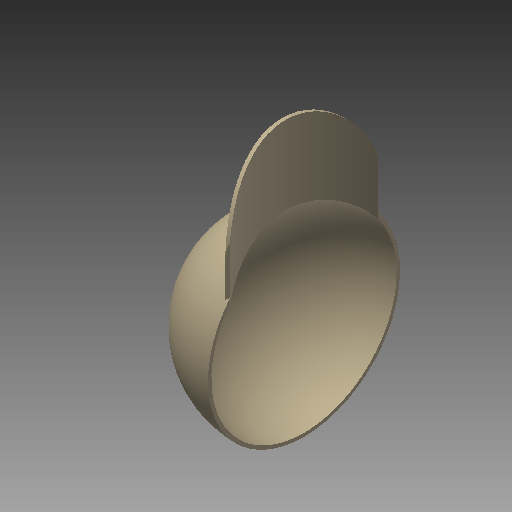
# Autodesk Inventor part: 3D HUMAN
Saved by Autodesk Inventor 2022 (Build 260153000, 153)
## iProperties
Category: PART
Part Number: 3D HUMAN
Document SubType Name: Modeling
Created: 2003-07-26
Designer: M.F.
Manufacturer: Standard
Standards Organization: Custom
Catalog Web Link: www.apollocanard.com
Density: 1 g/cm^3
Material: Generic
Appearance: Beige
Control State: 0
Master: False
Checked Out: False
Shininess: 64.0
Length Units: 11272
Angle Units: 11279
Time Units: 11290
Mass Units: 11286
Length Display Precision: 3
Angle Display Precision: 2
Compacted: True
Density: 0.0
Volumn: 0.0
Area: 0.0
PropertySet Name: Model Information
Title: iMan
Author: M.F.
Autodesk Inventor part; units mm, degrees
sketch "Sketch2" plane through (0, 0, 0) normal (0, 0, 1) x (1, 0, 0)
  line L0 (96.9814, 0) -> (100.5374, 0)
  arc A0 (100.5374, 0) -> (0, 100.5374) centre (0, 0) ccw
  line L1 (0, 100.5374) -> (0, 96.9814)
  arc A1 (96.9814, 0) -> (0, 96.9814) centre (0, 0) ccw
  dimension "d25" = 96.9814
  dimension "d26" = 3.556
  constraints: 4 end point, 4 point on circle, 2 centre point, 2 coincident, 2 point on line, 1 horizontal, 1 perpendicular
  measures "d25" radius of A1
  measures "d26" distance of L0.start L0.end
revolve "Revolution1" add sketch "Sketch2" angle 360 about axis through (0, 100.5374, 0) along (0, -1, 0)
ref_plane "Work Plane1" through (0, 0, 100.5374) normal (0, 0, 1) x (1, 0, 0)
ref_plane "Work Plane2" through (0, 0, 197.5188) normal (0, 0, 1) x (1, 0, 0)
sketch "Sketch4" plane through (0, 0, 197.5188) normal (0, 0, 1) x (1, 0, 0)
  line L0 (-96.9814, 0) -> (96.9814, 0) projected
  arc A0 (0, 19.3963) -> (-77.5851, 0) centre (0, -145.4721) ccw
  arc A1 (0, 22.9523) -> (-79.2585, 3.1376) centre (0, -145.4721) ccw
  line L1 (0, 19.3963) -> (0, 22.9523)
  line L2 (-79.2585, 3.1376) -> (-77.5851, 0)
  point P0 (0, 0)
  dimension "d30" = 19.3963
  dimension "d31" = 19.3963
  dimension "d32" = 3.556
  constraints: 5 point on circle, 4 end point, 2 centre point, 2 vertical alignment, 1 midpoint, 1 perpendicular, 1 point on line
  measures "d30" distance from line of A0.start L0
  measures "d31" distance of L0.start L2.end
  measures "d32" distance of L1.start L1.end
extrude "Extrusion1" add sketch "Sketch4" against normal up to next
mirror "Mirror1" about plane through (0, 19.3963, 197.5188) normal (1, 0, 0) of "Extrusion1"
sketch "Sketch5" plane through (0, 0, 197.5188) normal (0, 0, 1) x (1, 0, 0)
  arc A0 (77.5851, 0) -> (-77.5851, 0) centre (0, -145.4721) ccw projected
  line L0 (-77.5851, 0) -> (77.5851, 0)
  constraints: 2 end point, 1 horizontal
extrude "Extrusion2" cut sketch "Sketch5" against normal up to surface (197.5188 mm away)
sketch "Sketch6" plane through (0, 0, 0) normal (0, 1, 0) x (-1, 0, 0)
  arc A0 (79.2585, 97.8824) -> (-79.2585, 97.8824) centre (0, 97.8824) ccw
  spline S0 degree 3 poles (79.2585, 61.7739) (78.7898, 62.3626) (78.3161, 62.9424) (76.2018, 65.4662) (74.4059, 67.4387) (70.5529, 71.291) (68.4958, 73.1707) (64.2084, 76.7372) (61.9775, 78.4248) (57.4595, 81.5408) (55.1726, 82.9694) (49.2262, 86.3683) (45.2, 88.3377) (36.6968, 91.7804) (32.2196, 93.254) (23.0592, 95.6018) (18.3715, 96.4772) (9.0617, 97.6175) (4.4396, 97.8824) (0, 97.8824) knots 6.508033 6.508033 6.508033 6.508033 6.743552 6.743552 7.549615 7.549615 8.355677 8.355677 9.16174 9.16174 9.967802 9.967802 11.29968 11.29968 12.631559 12.631559 13.963437 13.963437 15.295315 15.295315 15.295315 15.295315 projected
  line L0 (79.2585, 197.5188) -> (79.2585, 61.7739) projected
  line L1 (-79.2585, 197.5188) -> (79.2585, 197.5188) projected
  line L2 (-79.2585, 197.5188) -> (-79.2585, 61.7739) projected
  spline S1 degree 3 poles (0, 97.8824) (-3.8082, 97.8824) (-7.782, 97.6875) (-15.8199, 96.8431) (-19.8839, 96.1936) (-27.8726, 94.4474) (-31.8002, 93.3501) (-39.3161, 90.7851) (-42.9045, 89.3173) (-50.7056, 85.6246) (-55.1538, 83.1048) (-63.6579, 77.2902) (-67.714, 73.9951) (-74.2398, 67.6766) (-76.8554, 64.7921) (-79.2585, 61.7739) knots 10.696449 10.696449 10.696449 10.696449 11.838902 11.838902 12.981356 12.981356 14.123809 14.123809 15.266262 15.266262 16.797921 16.797921 18.32958 18.32958 19.475682 19.475682 19.475682 19.475682 projected
  constraints: 2 point on circle, 2 point on line, 1 centre point, 1 coincident, 1 tangent
extrude "Extrusion3" cut sketch "Sketch6" along normal through all both and the other way through all contours A0 L2 L1 L0
ref_plane "Work Plane3" through (0, -12.9309, 0) normal (0, 1, 0) x (-1, 0, 0)
equation "\"d25\" = 0.5 * HEAD_TOP_WD"
equation "\"d30\" = 0.1 * HEAD_TOP_WD"
equation "\"d31\" = d30"
equation "\"d32\" = d26"
equation "\"d29\" = 0.5 * HEAD_TOP_WD"
equation "\"d39\" = -0.0666667 * HEAD_TOP_WD"
equation "\"HEAD_TOP_WD\" = 193.962833"
body "Solid1"
